PLATE_LV_SIDE (Autodesk Fusion 360 design; units mm, degrees)
Autodesk Fusion 360 part; units mm, degrees
sketch "Esquisse1" plane through (0, 0, 0) normal (0, 0, 1) x (1, 0, 0)
  line L0 (103, -50) -> (-103, -50)
  line L1 (-103, -50) -> (-103, 50)
  line L2 (-103, 50) -> (103, 50)
  line L3 (103, 50) -> (103, -50)
  line L4 (103, -50) -> (-103, 50) construction
  line L5 (-103, -50) -> (103, 50) construction
  line L6 (-100, -53) -> (100, -53)
  line L7 (100, -53) -> (100, 53)
  line L8 (100, 53) -> (-100, 53)
  line L9 (-100, 53) -> (-100, -53)
  line L10 (-100, -53) -> (100, 53) construction
  line L11 (100, -53) -> (-100, 53) construction
  dimension "d1" = 206
  dimension "d2" = 100
  dimension "d41" = 200
  dimension "d42" = 106
  constraint horizontal L0
  constraint perpendicular L0 L1
  constraint parallel L0 L2
  constraint parallel L1 L3
  constraint coincident L4 origin
  constraint coincident L5 origin
  constraint horizontal L6
  constraint perpendicular L6 L7
  constraint parallel L6 L8
  constraint parallel L7 L9
  constraint coincident L10 origin
  constraint coincident L11 origin
  measures "d1" distance of L1.end L2.end
  measures "d2" distance of L0.end L1.end
  measures "d41" distance of L7.end L8.end
  measures "d42" distance of L6.end L7.end
extrude "Extrusion1" add sketch "Esquisse1" along normal blind 3
sketch "Esquisse3" plane through (0, 0, 3) normal (0, 0, 1) x (-1, 0, 0)
  line L0 (100, -50) -> (103, -50)
  line L1 (103, -50) -> (103, 50)
  line L2 (103, 50) -> (100, 50)
  line L3 (-103, 50) -> (-103, -50)
  circle A0 centre (70, 0) radius 11.5
  circle A1 centre (37, 0) radius 10
  line L4 (-6.1, -21.1) -> (-93.9, -21.1)
  line L5 (-93.9, -21.1) -> (-93.9, 21.1)
  line L6 (-93.9, 21.1) -> (-6.1, 21.1)
  line L7 (-6.1, 21.1) -> (-6.1, -21.1)
  line L8 (-6.1, -21.1) -> (-93.9, 21.1) construction
  line L9 (-93.9, -21.1) -> (-6.1, 21.1) construction
  line L10 (-3.5, -27.5) -> (-96.5, -27.5)
  line L11 (-96.5, -27.5) -> (-96.5, 27.5)
  line L12 (-96.5, 27.5) -> (-3.5, 27.5)
  line L13 (-3.5, 27.5) -> (-3.5, -27.5)
  line L14 (-3.5, -27.5) -> (-96.5, 27.5) construction
  line L15 (-96.5, -27.5) -> (-3.5, 27.5) construction
  line L16 (103, 50) -> (103, -50)
  line L17 (-100, -50) -> (-100, -53)
  line L18 (-100, -53) -> (100, -53)
  line L19 (100, -53) -> (100, -50)
  line L20 (100, 50) -> (100, 53)
  line L21 (100, 53) -> (-100, 53)
  line L22 (-100, 53) -> (-100, 50)
  line L23 (-100, 50) -> (-103, 50)
  line L24 (-103, -50) -> (-100, -50)
  point P0 (-50, 0)
  point P1 (-50, 0)
  dimension "d15" = 23
  dimension "d19" = 50
  dimension "d22" = 33
  dimension "d23" = 20
  dimension "d26" = 3
  dimension "d27" = 100
  dimension "d28" = 50
  dimension "d30" = 87.8
  dimension "d31" = 42.2
  dimension "d32" = 50
  dimension "d34" = 93
  dimension "d35" = 55
  dimension "d40" = 66
  dimension "d43" = 50
  constraint horizontal L4
  constraint perpendicular L4 L5
  constraint parallel L4 L6
  constraint parallel L5 L7
  constraint coincident L8 P1
  constraint coincident L9 P1
  constraint horizontal L10
  constraint perpendicular L10 L11
  constraint parallel L10 L12
  constraint parallel L11 L13
  constraint coincident L14 P1
  constraint coincident L15 P1
  constraint coincident P1 P0
  measures "d15" diameter of A0
  measures "d19" distance of L0 A0.centre
  measures "d22" distance of L1 A0.centre
  measures "d23" diameter of A1
  measures "d26" distance of L0.start L0.end
  measures "d27" distance of L0.end L1.end
  measures "d28" distance of L0 A1.centre
  measures "d30" distance of L5.end L6.end
  measures "d31" distance of L4.end L5.end
  measures "d32" distance of L0 P1
  measures "d34" distance of L11.end L12.end
  measures "d35" distance of L10.end L11.end
  measures "d40" distance of A1.centre L16
  measures "d43" horizontal distance of origin P1
equation "d30 = 87.3 mm + 0.5 mm"
equation "d31 = 41.7 mm + 0.5 mm"
equation "d32 = d19"
